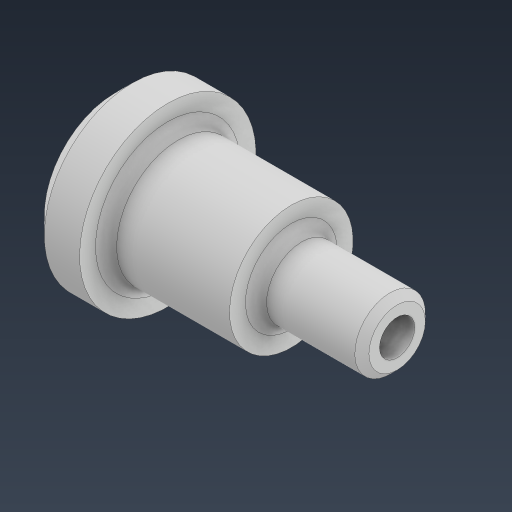
# Autodesk Inventor part: 3D Model
Saved by Autodesk Inventor 2024 (Build 280153000, 153)
## iProperties
Created: 2024-03-08
Part Number: 3D Model
Material: Genérico
Document SubType Name: Modeling
Designer: Administrator
Density: 1 g/cm^3
Appearance: Padrão
Author: Administrator
Autodesk Inventor part; units mm, degrees
ref_plane "YZ Plane" through (0, 0, 0) normal (1, 0, 0) x (0, 1, 0)
ref_plane "XZ Plane" through (0, 0, 0) normal (0, 1, 0) x (-1, 0, 0)
ref_plane "XY Plane" through (0, 0, 0) normal (0, 0, 1) x (1, 0, 0)
sketch "Esboço1" plane through (0, 0, 0) normal (0, 0, 1) x (1, 0, 0)
  line L0 (0, 0) -> (0, 25)
  line L1 (0, 25) -> (15, 25)
  line L2 (15, 25) -> (15, 17.5)
  line L3 (15, 17.5) -> (50, 17.5)
  line L4 (50, 17.5) -> (50, 10)
  line L5 (50, 10) -> (80, 10)
  line L6 (80, 10) -> (80, 0)
  line L7 (80, 0) -> (0, 0)
  dimension "d0" = 50
  dimension "d1" = 35
  dimension "d2" = 20
  dimension "d3" = 15
  dimension "d4" = 65
  dimension "d5" = 30
  constraints: 16 end point, 7 perpendicular, 1 vertical
  measures "d0" diameter of L1 L7
  measures "d1" diameter of L3 L7
  measures "d2" diameter of L5 L7
  measures "d3" distance between parallel lines of L2 L0
  measures "d4" distance between parallel lines of L2 L6
  measures "d5" distance between parallel lines of L6 L4
revolve "Revolução1" add sketch "Esboço1" angle 360 about axis through (80, 0, 0) along (-1, 0, 0)
fillet "Arredondamento1" radius 3 2 edges at (15, -17.5, 0) (50, -10, 0)
chamfer "Chanfro1" distance 2 angle 45 1 edges at (80, -10, 0)
chamfer "Chanfro2" distance 5 angle 45 1 edges at (0, -25, 0)
sketch "Esboço2" plane through (80, 0, 0) normal (1, 0, 0) x (0, 0, -1)
  circle A0 centre (0, 0) radius 10 projected
  constraints: 1 coincident
hole "Furo1" at (80, 0, 0) direction (-1, 0, 0) diameter 10 end through all
